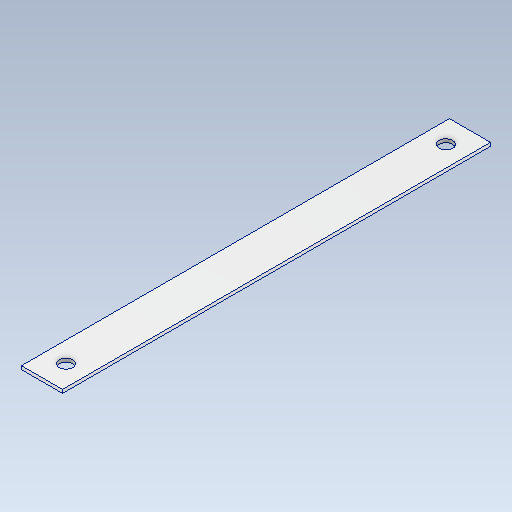
# Autodesk Inventor part: Barra fijación calefactor V2
Saved by Autodesk Inventor 2020 (Build 240168000, 168)
## iProperties
Created: 2020-06-08
Part Number: Barra fijación calefactor V2
Material: Aluminum 6061
Document SubType Name: Modeling
Designer: Bruno
Density: 2.7 g/cm^3
Appearance: Aluminum - Flat
Author: Bruno
Autodesk Inventor part; units mm, degrees
ref_plane "YZ Plane" through (0, 0, 0) normal (1, 0, 0) x (0, 1, 0)
ref_plane "XZ Plane" through (0, 0, 0) normal (0, 1, 0) x (-1, 0, 0)
ref_plane "XY Plane" through (0, 0, 0) normal (0, 0, 1) x (1, 0, 0)
sketch "Sketch1" plane through (0, 0, 0) normal (0, 1, 0) x (-1, 0, 0)
  line L0 (0, 0) -> (12, 0)
  line L1 (12, 0) -> (12, -125)
  line L2 (12, -125) -> (0, -125)
  line L3 (0, -125) -> (0, 0)
  circle A0 centre (6, -7) radius 2
  circle A1 centre (6, -118) radius 2
  dimension "d0" = 12
  dimension "d1" = 125
  dimension "d2" = 4
  dimension "d6" = 7
  dimension "d7" = 6
  dimension "d36" = 4
  dimension "d37" = 111
  dimension "d38" = 7
  constraints: 8 end point, 2 centre point, 2 parallel, 1 horizontal, 1 perpendicular, 1 vertical alignment
  measures "d0" distance of L1.end L2.end
  measures "d1" distance of L0.end L1.end
  measures "d2" diameter of A0
  measures "d6" distance from line of L0 A0.centre
  measures "d7" distance from line of L3 A0.centre
  measures "d36" diameter of A1
  measures "d37" distance of A0.centre A1.centre
  measures "d38" distance from line of L2 A1.centre
extrude "Extrusion1" add sketch "Sketch1" along normal blind 1
sketch "Sketch4" plane through (0, 1, 0) normal (0, 1, 0) x (1, 0, 0)
  circle A0 centre (-6, 118) radius 2 projected
  line L0 (-6, 118) -> (-6, 62.5) construction
  circle A1 centre (-6, 62.5) radius 55.5
  point P0 (0, 0)
  point P1 (-6, 3.7)
  dimension "d39" = 55.5
  constraints: 2 end point, 1 coincident, 1 vertical, 1 vertical alignment, 2 other
  measures "d39" distance of L0.start L0.end
body "Solid1"
